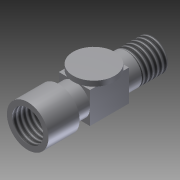
# Autodesk Inventor part: half inch flow valve
Saved by Autodesk Inventor 2011 (Build 150239000, 239)
## iProperties
Created: 2013-11-19
Part Number: half inch flow valve
Document SubType Name: Modeling
Designer: Devon
Density: 1 g/cm^3
Author: Devon
Autodesk Inventor part; units mm, degrees
ref_plane "YZ Plane" through (0, 0, 0) normal (1, 0, 0) x (0, 1, 0)
ref_plane "XZ Plane" through (0, 0, 0) normal (0, 1, 0) x (-1, 0, 0)
ref_plane "XY Plane" through (0, 0, 0) normal (0, 0, 1) x (1, 0, 0)
sketch "Sketch1" plane through (0, 0, 0) normal (0, 0, 1) x (1, 0, 0)
  circle A0 centre (0, 0) radius 6.35
  circle A1 centre (0, 0) radius 7.62
  dimension "d0" = 12.7
  dimension "d1" = 15.24
  constraints: 2 centre point, 2 coincident
  measures "d0" diameter of A0
  measures "d1" diameter of A1
extrude "Extrusion1" add sketch "Sketch1" along normal blind 19.05
thread "Thread1" size "5/8-11 UNC" class "2A" standard "ANSI Unified Screw Threads" length 12.7
sketch "Sketch3" plane through (0, 0, 19.05) normal (0, 0, 1) x (1, 0, 0)
  circle A0 centre (0, 0) radius 6.35 projected
  line L0 (-7.62, 7.62) -> (7.62, 7.62)
  line L1 (7.62, 7.62) -> (7.62, -7.62)
  line L2 (7.62, -7.62) -> (-7.62, -7.62)
  line L3 (-7.62, -7.62) -> (-7.62, 7.62)
  constraints: 8 end point, 2 parallel, 1 horizontal, 1 perpendicular
extrude "Extrusion2" add sketch "Sketch3" along normal blind 19.05
sketch "Sketch4" plane through (0, 0, 38.1) normal (0, 0, 1) x (1, 0, 0)
  circle A0 centre (0, 0) radius 6.35 projected
  circle A1 centre (0, 0) radius 6.35
  circle A2 centre (0, 0) radius 7.62
  constraints: 2 centre point, 2 coincident, 1 concentric
extrude "Extrusion3" add sketch "Sketch4" along normal blind 7.62
sketch "Sketch5" plane through (0, 0, 45.72) normal (0, 0, 1) x (1, 0, 0)
  circle A0 centre (0, 0) radius 7.62 projected
  circle A1 centre (0, 0) radius 7.62
  circle A2 centre (0, 0) radius 10.16
  dimension "d10" = 20.32
  constraints: 2 centre point, 1 coincident, 1 concentric
  measures "d10" diameter of A2
extrude "Extrusion4" add sketch "Sketch5" along normal blind 15.24
sketch "Sketch6" plane through (0, 7.62, 19.05) normal (0, 1, 0) x (1, 0, 0)
  circle A0 centre (0, -9.525) radius 10.16
  point P0 (0, 19.05)
  dimension "d13" = 20.32
  constraints: 1 centre point
  measures "d13" diameter of A0
extrude "Extrusion5" add sketch "Sketch6" along normal blind 2.54
thread "Thread2" size "5/8-11 UNC" class "2B" standard "ANSI Unified Screw Threads" length 25.4
body "Solid1"
